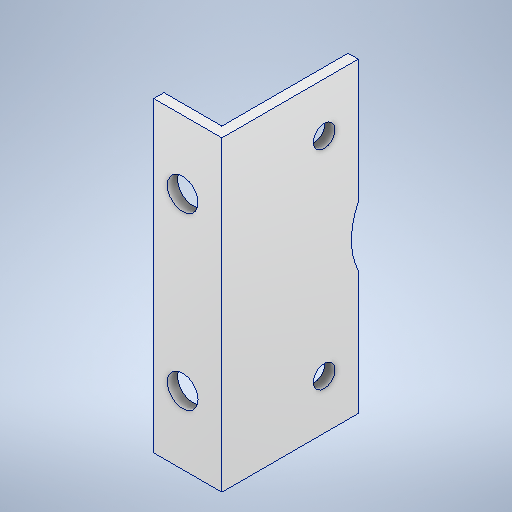
# Autodesk Inventor part: x_bracket_stepper
Saved by Autodesk Inventor 2025 (Build 290162000, 162)
## iProperties
Created: 2024-04-25
Part Number: x_bracket_stepper
Material: Hliník 6061
Document SubType Name: Modeling
Designer: rader
Density: 2.7 g/cm^3
Appearance: Hliník – plochý
Author: rader
Autodesk Inventor part; units mm, degrees
ref_plane "YZ Plane" through (0, 0, 0) normal (1, 0, 0) x (0, 1, 0)
ref_plane "XZ Plane" through (0, 0, 0) normal (0, 1, 0) x (-1, 0, 0)
ref_plane "XY Plane" through (0, 0, 0) normal (0, 0, 1) x (1, 0, 0)
sketch "Náčrt1" plane through (0, 0, 0) normal (0, 0, 1) x (1, 0, 0)
  line L0 (-10, 0) -> (0, 0)
  line L1 (0, 0) -> (0, 20)
  line L2 (0, 20) -> (-1.5, 20)
  line L3 (-1.5, 20) -> (-1.5, 1.5)
  line L4 (-1.5, 1.5) -> (-10, 1.5)
  line L5 (-10, 1.5) -> (-10, 0)
  line L6 (-12, 0) -> (2, 0) projected
  line L7 (0, 24) -> (0, -4) projected
  point P0 (0, 0)
  dimension "d0" = 20
  dimension "d1" = 10
  dimension "d2" = 1.5
  dimension "d3" = 1.5
  constraints: 12 end point, 5 perpendicular, 3 collinear, 1 horizontal
  measures "d0" distance of L0.end L1.end
  measures "d1" distance of L0.start L0.end
  measures "d2" distance between parallel lines of L3 L1
  measures "d3" distance between parallel lines of L4 L0
extrude "Vysunutí1" add sketch "Náčrt1" along normal mid plane 45
sketch "Náčrt2" plane through (-10, 1.5, 22.5) normal (0, 1, 0) x (1, 0, 0)
  line L0 (0, 0) -> (0, 45) projected
  line L1 (8.5, 0) -> (0, 0) projected
  line L2 (8.5, 45) -> (8.5, 0) projected
  line L3 (0, 45) -> (8.5, 45) projected
  point P0 (10, 22.5)
  point P1 (4.25, 35)
  point P2 (4.25, 10)
  point P3 (4.25, 0)
  dimension "d6" = 4.25
  dimension "d7" = 4.25
  dimension "d8" = 25
  dimension "d9" = 10
  constraints: 1 midpoint
  measures "d6" distance from line of L0 point (4.25, 10)
  measures "d7" distance from line of L0 point (4.25, 35)
  measures "d8" distance of point (4.25, 10) point (4.25, 35)
  measures "d9" distance of point (4.25, 0) point (4.25, 10)
hole "Díra1" at (-5.75, 1.5, -12.5) at (-5.75, 1.5, 12.5) direction (0, -1, 0) diameter 4.5 end through all
sketch "Náčrt5" plane through (0, 0, 22.5) normal (1, 0, 0) x (0, 0, -1)
  line L0 (45, 20) -> (0, 20) projected
  line L1 (0, 0) -> (0, 20) projected
  line L2 (45, 0) -> (0, 0) projected
  line L3 (45, 20) -> (45, 0) projected
  line L4 (22.5, 0) -> (22.5, 47.1534) construction
  point P0 (22.5, 20)
  point P1 (37.75, 15)
  point P2 (7.25, 15)
  dimension "d41" = 30.5
  dimension "d42" = 5
  dimension "d43" = 47.1534
  constraints: 2 end point, 1 midpoint, 1 symmetric about line, 1 vertical
  measures "d41" distance of point (7.25, 15) point (37.75, 15)
  measures "d42" distance from line of L0 point (37.75, 15)
  measures "d43" distance of L4.start L4.end
hole "Díra4" at (0, 15, -15.25) at (0, 15, 15.25) direction (-1, 0, 0) diameter 3.2 end through all
sketch "Náčrt6" plane through (0, 0, 22.5) normal (1, 0, 0) x (0, 0, -1)
  line L0 (22.5, 0) -> (22.5, 40) construction
  circle A0 centre (22.5, 29) radius 10
  point P0 (22.5, 19)
  point P1 (22.5, 20)
  dimension "d52" = 20
  dimension "d51" = 40
  dimension "d53" = 1
  constraints: 2 end point, 2 point on line, 1 midpoint, 1 vertical, 1 vertical alignment, 2 other
  measures "d51" distance of L0.start L0.end
  measures "d53" distance of point (22.5, 20) point (22.5, 19)
extrude "Vysunutí2" cut sketch "Náčrt6" against normal through all
